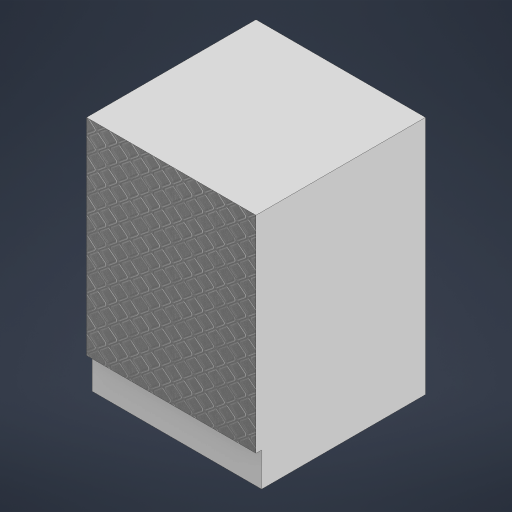
# Autodesk Inventor part: Mobile lavastoviglie
Saved by Autodesk Inventor 2024.2 (Build 282272000, 272)
## iProperties
Created: 2025-08-13
Part Number: Mobile lavastoviglie
Material: Generic
Document SubType Name: Modeling
Designer: Luca
Density: 1 g/cm^3
Appearance: Default
Author: Luca
Autodesk Inventor part; units mm, degrees
ref_plane "YZ Plane" through (0, 0, 0) normal (1, 0, 0) x (0, 1, 0)
ref_plane "XZ Plane" through (0, 0, 0) normal (0, 1, 0) x (-1, 0, 0)
ref_plane "XY Plane" through (0, 0, 0) normal (0, 0, 1) x (1, 0, 0)
sketch "Sketch1" plane through (0, 0, 0) normal (0, 1, 0) x (-1, 0, 0)
  line L0 (300, 0) -> (-300, 0)
  line L1 (-300, 0) -> (-300, 600)
  line L2 (-300, 600) -> (300, 600)
  line L3 (300, 600) -> (300, 0)
  point P0 (0, 0)
  point P1 (0, 0)
  dimension "d0" = 600
  dimension "d1" = 600
  constraints: 8 end point, 2 parallel, 1 coincident, 1 horizontal, 1 midpoint, 1 perpendicular
  measures "d0" distance of L1.end L2.end
  measures "d1" distance of L0.end L1.end
extrude "Extrusion1" add sketch "Sketch1" along normal blind 850
sketch "Sketch3" plane through (-300, 0, 600) normal (0, 0, 1) x (1, 0, 0)
  line L0 (0, 0) -> (600, 0) projected
  line L1 (600, 0) -> (600, 850) projected
  line L2 (0, 0) -> (600, 0)
  line L3 (600, 0) -> (600, 120)
  line L4 (600, 120) -> (0, 120)
  line L5 (0, 120) -> (0, 0)
  point P0 (300, 0)
  dimension "d9" = 120
  constraints: 8 end point, 2 parallel, 1 horizontal, 1 perpendicular, 1 point on line
  measures "d9" distance of L3.end L2.end
extrude "Extrusion3" cut sketch "Sketch3" against normal blind 20
body "Solid1"
